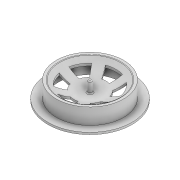
# Autodesk Inventor part: mask_breath_bottom
Saved by Autodesk Inventor 2021 (Build 250183000, 183)
## iProperties
Created: 2020-04-12
Part Number: mask_breath_bottom
Material: Generic
Document SubType Name: Modeling
Designer: Muchiri John
Density: 1 g/cm^3
Appearance: Default
Author: Muchiri John
Autodesk Inventor part; units mm, degrees
ref_plane "YZ Plane" through (0, 0, 0) normal (1, 0, 0) x (0, 1, 0)
ref_plane "XZ Plane" through (0, 0, 0) normal (0, 1, 0) x (-1, 0, 0)
ref_plane "XY Plane" through (0, 0, 0) normal (0, 0, 1) x (1, 0, 0)
sketch "Sketch1" plane through (0, 0, 0) normal (0, 0, 1) x (1, 0, 0)
  line L0 (7.1818, 17.8522) -> (11.3818, 17.8522)
  line L1 (12.3818, 16.8522) -> (7.1818, 16.8522)
  line L2 (7.1818, 16.8522) -> (7.1818, 17.8522)
  line L3 (11.3818, 25.8522) -> (11.3818, 17.8522)
  line L4 (28.1818, 25.8522) -> (28.1818, 19.3327)
  line L5 (26.6739, 19.3327) -> (28.1818, 19.3327)
  line L6 (12.3818, 16.8522) -> (12.3818, 23.7208)
  line L7 (11.3818, 25.8522) -> (12.6715, 25.8522)
  line L8 (28.1818, 25.8522) -> (27.7018, 25.8522)
  line L9 (27.2018, 25.3522) -> (27.2018, 20.8252)
  arc A0 (13.0269, 25.7039) -> (26.7229, 20.3257) centre (25.9545, 38.4967) ccw
  arc A1 (13.2079, 24.0999) -> (26.6739, 19.3327) centre (26.0829, 39.0659) ccw
  arc A2 (27.7018, 25.8522) -> (27.2018, 25.3522) centre (27.7018, 25.3522) ccw
  arc A3 (13.0269, 25.7039) -> (12.6715, 25.8522) centre (12.6715, 25.3522) ccw
  arc A4 (13.2079, 24.0999) -> (12.3818, 23.7208) centre (12.8818, 23.7208) ccw
  arc A5 (26.7229, 20.3257) -> (27.2018, 20.8252) centre (26.7018, 20.8252) ccw
  point P0 (12.3818, 24.8522)
  point P1 (12.8818, 25.8522)
  point P2 (27.2018, 25.8522)
  point P3 (27.2018, 20.3522)
  dimension "d20" = 21
  dimension "d21" = 15.8
  dimension "d22" = 1
  dimension "d40" = 1
  dimension "d47" = 1.5
  dimension "d48" = 0.98
  dimension "d49" = 5.5
  dimension "d50" = 0.5
  constraints: 20 end point, 15 point on circle, 8 tangent, 6 centre point, 5 point on line, 4 horizontal, 3 equal radius, 1 parallel, 1 perpendicular, 1 vertical
  measures "d20" distance between parallel lines of L4 L2
  measures "d21" distance between parallel lines of L6 L4
  measures "d22" distance between parallel lines of L3 L6
  measures "d40" distance between parallel lines of L0 L1
  measures "d47" distance of L3.start point (12.882, 25.852)
  measures "d48" distance of L4.start point (27.202, 25.852)
  measures "d49" distance of point (27.202, 25.852) point (27.202, 20.352)
  measures "d50" radius of A2
revolve "Mask_Breath_Bottom" add sketch "Sketch1" angle 360 about axis through (28.1818, 25.8522, 0) along (0, -1, 0)
sketch "Sketch6" plane through (28.1818, 25.8522, 0) normal (0, 1, 0) x (1, 0, 0)
  circle A0 centre (0, 0) radius 0.48 projected
  arc A1 (-3.9463, -12.3865) -> (4.4814, -12.2031) centre (0, 0) ccw
  arc A2 (-1.9198, -7.7662) -> (1.9198, -7.7662) centre (0, 0) ccw
  line L0 (1.9198, -7.7662) -> (4.4814, -12.2031)
  line L1 (1.9198, -7.7662) -> (7.8134, -7.7662) construction
  line L2 (-1.9198, -7.7662) -> (-3.9463, -12.3865)
  arc A3 (-12.7002, -2.7757) -> (-8.3275, -9.9826) centre (0, 0) ccw
  arc A4 (-7.6857, -2.2205) -> (-5.7659, -5.5457) centre (0, 0) ccw
  line L3 (-5.7659, -5.5457) -> (-8.3275, -9.9826)
  line L4 (-5.7659, -5.5457) -> (-2.8191, -10.6497) construction
  line L5 (-7.6857, -2.2205) -> (-12.7002, -2.7757)
  arc A5 (-8.7539, 9.6109) -> (-12.809, 2.2205) centre (0, 0) ccw
  arc A6 (-5.7659, 5.5457) -> (-7.6857, 2.2205) centre (0, 0) ccw
  line L6 (-7.6857, 2.2205) -> (-12.809, 2.2205)
  line L7 (-7.6857, 2.2205) -> (-10.6324, -2.8835) construction
  line L8 (-5.7659, 5.5457) -> (-8.7539, 9.6109)
  arc A7 (3.9463, 12.3865) -> (-4.4814, 12.2031) centre (0, 0) ccw
  arc A8 (1.9198, 7.7662) -> (-1.9198, 7.7662) centre (0, 0) ccw
  line L9 (-1.9198, 7.7662) -> (-4.4814, 12.2031)
  line L10 (-1.9198, 7.7662) -> (-7.8134, 7.7662) construction
  line L11 (1.9198, 7.7662) -> (3.9463, 12.3865)
  arc A9 (12.7002, 2.7757) -> (8.3275, 9.9826) centre (0, 0) ccw
  arc A10 (7.6857, 2.2205) -> (5.7659, 5.5457) centre (0, 0) ccw
  line L12 (5.7659, 5.5457) -> (8.3275, 9.9826)
  line L13 (5.7659, 5.5457) -> (2.8191, 10.6497) construction
  line L14 (7.6857, 2.2205) -> (12.7002, 2.7757)
  arc A11 (8.7539, -9.6109) -> (12.809, -2.2205) centre (0, 0) ccw
  arc A12 (5.7659, -5.5457) -> (7.6857, -2.2205) centre (0, 0) ccw
  line L15 (7.6857, -2.2205) -> (12.809, -2.2205)
  line L16 (7.6857, -2.2205) -> (10.6324, 2.8835) construction
  line L17 (5.7659, -5.5457) -> (8.7539, -9.6109)
  dimension "d51" = 26
  dimension "d52" = 16
  dimension "d53" = 60
  dimension "d56" = 360
  constraints: 36 end point, 24 point on circle, 12 centre point, 9 coincident, 1 horizontal, 71 other
  measures "d51" diameter of A1
  measures "d52" diameter of A2
  measures "d53" angle of L0 L1
extrude "Extrusion2" cut sketch "Sketch6" against normal blind 10 contours L2 A2 L0 A1 | L5 A4 L3 A3 | L8 A6 L6 A5 | L11 A8 L9 A7 | L14 A10 L12 A9 | L17 A12 L15 A11
body "Solid1"
